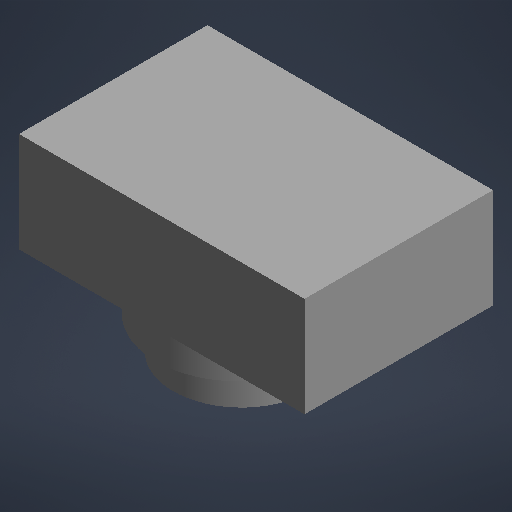
# Autodesk Inventor part: test_two_sketch_planes_cad_model
Saved by Autodesk Inventor 2026 (Build 300175050, 175E)
## iProperties
Part Number: test_two_sketch_planes_cad_model
Material: Generic
Document SubType Name: Modeling
Designer: Administrator
Appearance: Default
Author: Administrator
Autodesk Inventor part; units mm, degrees
ref_plane "Work Plane1" through (0, 0, 0) normal (0, 0, 1) x (1, 0, 0)
sketch "Sketch1" plane through (0, 0, 0) normal (0, 0, 1) x (1, 0, 0)
  line L0 (-6.5, 6.3) -> (3.5, 6.3)
  line L1 (3.5, 6.3) -> (3.5, 6)
  line L2 (3.5, 6) -> (3.5, 4.6)
  line L3 (3.5, 2.8) -> (3.5, 4.6)
  line L4 (-6.5, 2.8) -> (3.5, 2.8)
  line L5 (-6.5, 6.3) -> (-6.5, 2.8)
  constraints: 12 end point
extrude "Extrusion1" add sketch "Sketch1" along normal blind 6.6
ref_plane "Work Plane2" through (-1.5, 2.8, 3.3) normal (0, -1, 0) x (1, 0, 0)
sketch "Sketch2" plane through (-1.5, 2.8, 3.3) normal (0, -1, 0) x (1, 0, 0)
  circle A0 centre (-0.3, 0.3) radius 2.9
  constraints: 1 centre point
extrude "Extrusion2" add sketch "Sketch2" along normal blind 1.1 separate body
ref_plane "Work Plane3" through (-1.7, 1.7, 3.6) normal (0, -1, 0) x (1, 0, 0)
sketch "Sketch3" plane through (-1.7, 1.7, 3.6) normal (0, -1, 0) x (1, 0, 0)
  circle A0 centre (0, 0) radius 2.4
  constraints: 1 centre point
extrude "Extrusion3" add sketch "Sketch3" along normal blind 1.1 separate body
body "Solid1"
body "Solid2"
body "Solid3"
